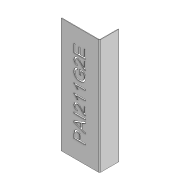
# Autodesk Inventor part: Laterales
Saved by Autodesk Inventor 2021 (Build 250183000, 183)
## iProperties
Created: 2021-04-18
Part Number: Laterales
Material: Genérico
Document SubType Name: Chapa
Designer: carlo
Density: 1 g/cm^3
Sheet Metal Rule: Por defecto_mm
Appearance: Valor por defecto
Author: carlo
Autodesk Inventor part; units mm, degrees
ref_plane "YZ Plane" through (0, 0, 0) normal (1, 0, 0) x (0, 1, 0)
ref_plane "XZ Plane" through (0, 0, 0) normal (0, 1, 0) x (-1, 0, 0)
ref_plane "XY Plane" through (0, 0, 0) normal (0, 0, 1) x (1, 0, 0)
sketch "Boceto1" plane through (0, 0, 0) normal (0, 0, 1) x (1, 0, 0)
  line L0 (0, 0) -> (200, 0)
  line L1 (200, 0) -> (200, 600)
  line L2 (200, 600) -> (0, 600)
  line L3 (0, 600) -> (0, 0)
  dimension "d0" = 200
  dimension "d1" = 600
  measures "d0" distance of L2.end L1.end
  measures "d1" distance of L1.end L0.end
extrude "Placa1" add sketch "Boceto1" along normal blind 3
sketch "Boceto2" plane through (197, 600, 3) normal (1, 0, 0) x (0, 1, 0)
  line L0 (-600, 0) -> (0, 0)
  line L1 (0, 0) -> (0, 100)
  line L2 (0, 100) -> (-600, 100)
  line L3 (-600, 100) -> (-600, 0)
  constraints: 6 end point, 1 horizontal, 1 perpendicular, 1 vertical
edge flange "Pestaña1" height 100 angle -90 thickness 3 bend radius 3 thickness toward (1, 0, 0) relief straight relief width 3 relief depth 1.5 edges at (200, 300, 3) wall of the first edge with corners at (197, 0, 3) (197, 600, 3) (197, 600, -97) (197, 0, -97)
bend "Doblez1"
corner "Esquina1"
sketch "Boceto3" plane through (0, 0, 3) normal (0, 0, 1) x (1, 0, 0)
  line L0 (65.3644, 82.3487) -> (65.3644, 522.9888) construction
  line L1 (65.3644, 522.9888) -> (130.6275, 522.9888) construction
  line L2 (130.6275, 522.9888) -> (130.6275, 82.3487) construction
  line L3 (130.6275, 82.3487) -> (65.3644, 82.3487) construction
  line L4 (0, 0) -> (0, 600) projected
  line L5 (194, 0) -> (0, 0) projected
  line L6 (0, 600) -> (194, 600) projected
  line L7 (126.4162, 88.7968) -> (66.4162, 88.7968)
  line L8 (66.4162, 88.7968) -> (66.4162, 111.434)
  spline S0 degree 2 poles (66.4162, 111.434) (66.4162, 117.4249) (67.0107, 120.5804) knots 0 0 0 1 1 1
  spline S1 degree 2 poles (67.0107, 120.5804) (67.7424, 125.0163) (71.8583, 130.9615) (79.3125, 134.62) (83.7942, 134.62) knots 0 0 0 1 2 3 3 3
  spline S2 degree 2 poles (83.7942, 134.62) (91.4314, 134.62) (102.0412, 124.8791) (102.0412, 112.1657) knots 0 0 0 1 2 2 2
  line L9 (102.0412, 112.1657) -> (102.0412, 96.7541)
  line L10 (102.0412, 96.7541) -> (126.4162, 96.7541)
  line L11 (126.4162, 96.7541) -> (126.4162, 88.7968)
  line L12 (94.9528, 96.7541) -> (94.9528, 112.2572)
  spline S3 degree 2 poles (94.9528, 112.2572) (94.9528, 119.9859) (89.2363, 126.434) (84.0229, 126.434) knots 0 0 0 1 2 2 2
  spline S4 degree 2 poles (84.0229, 126.434) (80.2729, 126.434) (74.8766, 122.6383) (74.0534, 119.5285) knots 0 0 0 1 2 2 2
  spline S5 degree 2 poles (74.0534, 119.5285) (73.5046, 117.5163) (73.5046, 112.12) knots 0 0 0 1 1 1
  line L13 (73.5046, 112.12) -> (73.5046, 96.7541)
  line L14 (73.5046, 96.7541) -> (94.9528, 96.7541)
  line L15 (126.4162, 138.1871) -> (66.4162, 161.2359)
  line L16 (66.4162, 161.2359) -> (66.4162, 169.8334)
  line L17 (66.4162, 169.8334) -> (126.4162, 194.3456)
  line L18 (126.4162, 194.3456) -> (126.4162, 185.2907)
  line L19 (126.4162, 185.2907) -> (108.2607, 178.3395)
  line L20 (108.2607, 178.3395) -> (108.2607, 153.1871)
  line L21 (108.2607, 153.1871) -> (126.4162, 146.6017)
  line L22 (126.4162, 146.6017) -> (126.4162, 138.1871)
  line L23 (101.8125, 155.4737) -> (101.8125, 175.87)
  line L24 (101.8125, 175.87) -> (85.1662, 169.559)
  spline S6 degree 2 poles (85.1662, 169.559) (77.5747, 166.7237) (72.7272, 165.3517) knots 0 0 0 1 1 1
  spline S7 degree 2 poles (72.7272, 165.3517) (78.4894, 164.1627) (84.2058, 162.1048) knots 0 0 0 1 1 1
  line L25 (84.2058, 162.1048) -> (101.8125, 155.4737)
  line L26 (126.4162, 202.0285) -> (66.4162, 202.0285)
  line L27 (66.4162, 202.0285) -> (66.4162, 209.9859)
  line L28 (66.4162, 209.9859) -> (126.4162, 209.9859)
  line L29 (126.4162, 209.9859) -> (126.4162, 202.0285)
  line L30 (119.3278, 259.6505) -> (126.4162, 259.6505)
  line L31 (126.4162, 259.6505) -> (126.4162, 220.0011)
  spline S8 degree 2 poles (126.4162, 220.0011) (123.7638, 219.9096) (121.2942, 220.87) knots 0 0 0 1 1 1
  spline S9 degree 2 poles (121.2942, 220.87) (117.2241, 222.3791) (109.404, 229.056) (104.2363, 235.367) knots 0 0 0 1 2 2 2
  spline S10 degree 2 poles (104.2363, 235.367) (96.1875, 245.1078) (86.8583, 251.9676) (82.651, 251.9676) knots 0 0 0 1 2 2 2
  spline S11 degree 2 poles (82.651, 251.9676) (78.2607, 251.9676) (72.2699, 245.7023) (72.2699, 240.6718) knots 0 0 0 1 2 2 2
  spline S12 degree 2 poles (72.2699, 240.6718) (72.2699, 235.367) (78.6723, 229.0102) (84.2973, 228.9645) knots 0 0 0 1 2 2 2
  line L32 (84.2973, 228.9645) -> (83.5199, 221.373)
  spline S13 degree 2 poles (83.5199, 221.373) (75.0595, 222.1505) (66.1875, 232.3029) (66.1875, 240.8548) knots 0 0 0 1 2 2 2
  spline S14 degree 2 poles (66.1875, 240.8548) (66.1875, 249.498) (75.7455, 259.559) (82.8339, 259.559) knots 0 0 0 1 2 2 2
  spline S15 degree 2 poles (82.8339, 259.559) (86.4467, 259.559) (93.3979, 256.6322) (101.0808, 249.7724) (107.8034, 241.8609) knots 0 0 0 1 2 3 3 3
  spline S16 degree 2 poles (107.8034, 241.8609) (113.3369, 235.2298) (117.3156, 231.4798) (119.3278, 230.245) knots 0 0 0 1 2 2 2
  line L33 (119.3278, 230.245) -> (119.3278, 259.6505)
  line L34 (126.4162, 295.2755) -> (126.4162, 287.9127)
  line L35 (126.4162, 287.9127) -> (79.4955, 287.9127)
  spline S17 degree 2 poles (79.4955, 287.9127) (82.0107, 285.2602) (87.0869, 276.617) (88.3674, 273.1871) knots 0 0 0 1 2 2 2
  line L36 (88.3674, 273.1871) -> (81.2333, 273.1871)
  spline S18 degree 2 poles (81.2333, 273.1871) (78.3522, 279.3609) (70.0747, 288.5987) (66.1875, 290.5194) knots 0 0 0 1 2 2 2
  line L37 (66.1875, 290.5194) -> (66.1875, 295.2755)
  line L38 (66.1875, 295.2755) -> (126.4162, 295.2755)
  line L39 (126.4162, 341.8761) -> (126.4162, 334.5133)
  line L40 (126.4162, 334.5133) -> (79.4955, 334.5133)
  spline S19 degree 2 poles (79.4955, 334.5133) (82.0107, 331.8609) (87.0869, 323.2176) (88.3674, 319.7877) knots 0 0 0 1 2 2 2
  line L41 (88.3674, 319.7877) -> (81.2333, 319.7877)
  spline S20 degree 2 poles (81.2333, 319.7877) (78.3522, 325.9615) (70.0747, 335.1993) (66.1875, 337.12) knots 0 0 0 1 2 2 2
  line L42 (66.1875, 337.12) -> (66.1875, 341.8761)
  line L43 (66.1875, 341.8761) -> (126.4162, 341.8761)
  line L44 (102.9101, 391.8609) -> (95.8217, 391.8609)
  line L45 (95.8217, 391.8609) -> (95.8217, 417.242)
  line L46 (95.8217, 417.242) -> (118.0473, 417.242)
  spline S21 degree 2 poles (118.0473, 417.242) (122.7119, 411.3883) (127.4223, 398.9493) (127.4223, 392.4096) knots 0 0 0 1 2 2 2
  spline S22 degree 2 poles (127.4223, 392.4096) (127.4223, 383.5834) (119.8308, 369.1322) (105.5168, 361.7694) (96.6906, 361.7694) knots 0 0 0 1 2 3 3 3
  spline S23 degree 2 poles (96.6906, 361.7694) (87.9101, 361.7694) (72.7272, 369.0865) (65.3644, 382.8517) (65.3644, 391.8151) knots 0 0 0 1 2 3 3 3
  spline S24 degree 2 poles (65.3644, 391.8151) (65.3644, 398.309) (69.5717, 408.8273) (77.1174, 414.7724) (83.1997, 416.3273) knots 0 0 0 1 2 3 3 3
  line L47 (83.1997, 416.3273) -> (85.1662, 409.1932)
  spline S25 degree 2 poles (85.1662, 409.1932) (80.593, 407.8212) (75.3339, 403.8426) (72.1784, 396.3883) (72.1784, 391.8609) knots 0 0 0 1 2 3 3 3
  spline S26 degree 2 poles (72.1784, 391.8609) (72.1784, 386.4188) (75.4711, 378.4615) (80.9131, 373.6139) (84.1144, 372.242) knots 0 0 0 1 2 3 3 3
  spline S27 degree 2 poles (84.1144, 372.242) (89.6936, 369.9554) (96.1875, 369.9554) knots 0 0 0 1 1 1
  spline S28 degree 2 poles (96.1875, 369.9554) (104.1906, 369.9554) (115.029, 375.4889) (120.2424, 386.0529) (120.2424, 391.9523) knots 0 0 0 1 2 3 3 3
  spline S29 degree 2 poles (120.2424, 391.9523) (120.2424, 397.12) (116.2638, 406.9523) (114.0229, 409.4676) knots 0 0 0 1 2 2 2
  line L48 (114.0229, 409.4676) -> (102.9101, 409.4676)
  line L49 (102.9101, 409.4676) -> (102.9101, 391.8609)
  line L50 (119.3278, 464.6657) -> (126.4162, 464.6657)
  line L51 (126.4162, 464.6657) -> (126.4162, 425.0163)
  spline S30 degree 2 poles (126.4162, 425.0163) (123.7638, 424.9249) (121.2942, 425.8852) knots 0 0 0 1 1 1
  spline S31 degree 2 poles (121.2942, 425.8852) (117.2241, 427.3944) (109.404, 434.0712) (104.2363, 440.3822) knots 0 0 0 1 2 2 2
  spline S32 degree 2 poles (104.2363, 440.3822) (96.1875, 450.123) (86.8583, 456.9828) (82.651, 456.9828) knots 0 0 0 1 2 2 2
  spline S33 degree 2 poles (82.651, 456.9828) (78.2607, 456.9828) (72.2699, 450.7176) (72.2699, 445.6871) knots 0 0 0 1 2 2 2
  spline S34 degree 2 poles (72.2699, 445.6871) (72.2699, 440.3822) (78.6723, 434.0255) (84.2973, 433.9798) knots 0 0 0 1 2 2 2
  line L52 (84.2973, 433.9798) -> (83.5199, 426.3883)
  spline S35 degree 2 poles (83.5199, 426.3883) (75.0595, 427.1657) (66.1875, 437.3182) (66.1875, 445.87) knots 0 0 0 1 2 2 2
  spline S36 degree 2 poles (66.1875, 445.87) (66.1875, 454.5133) (75.7455, 464.5743) (82.8339, 464.5743) knots 0 0 0 1 2 2 2
  spline S37 degree 2 poles (82.8339, 464.5743) (86.4467, 464.5743) (93.3979, 461.6474) (101.0808, 454.7877) (107.8034, 446.8761) knots 0 0 0 1 2 3 3 3
  spline S38 degree 2 poles (107.8034, 446.8761) (113.3369, 440.245) (117.3156, 436.495) (119.3278, 435.2602) knots 0 0 0 1 2 2 2
  line L53 (119.3278, 435.2602) -> (119.3278, 464.6657)
  line L54 (126.4162, 475.7328) -> (66.4162, 475.7328)
  line L55 (66.4162, 475.7328) -> (66.4162, 519.1779)
  line L56 (66.4162, 519.1779) -> (73.5046, 519.1779)
  line L57 (73.5046, 519.1779) -> (73.5046, 483.6901)
  line L58 (73.5046, 483.6901) -> (91.843, 483.6901)
  line L59 (91.843, 483.6901) -> (91.843, 516.9371)
  line L60 (91.843, 516.9371) -> (98.9314, 516.9371)
  line L61 (98.9314, 516.9371) -> (98.9314, 483.6901)
  line L62 (98.9314, 483.6901) -> (119.3278, 483.6901)
  line L63 (119.3278, 483.6901) -> (119.3278, 520.5499)
  line L64 (119.3278, 520.5499) -> (126.4162, 520.5499)
  line L65 (126.4162, 520.5499) -> (126.4162, 475.7328)
  constraints: 1 parallel, 2 other
emboss "Repujado1" sketch "Boceto3" operation cut depth 3 direction (0, 0, -1)
equation "\"d2\" = Grosor"
equation "\"d3\" = Anchura_desahogo_plegado"
equation "\"d4\" = Profundidad_desahogo_plegado"
equation "\"d5\" = Remanente_mínimo"
equation "\"d6\" = Radiodetransición"
equation "\"d9\" = Radio_pliegue"
equation "\"d10\" = Tamaño_destalonado"
equation "\"d11\" = TamañoSeparación"
equation "\"d12\" = Tamaño_de_radio_de_Jacobi"
equation "\"Radio_pliegue\" = Grosor"
equation "\"Anchura_desahogo_plegado\" = Grosor"
equation "\"Profundidad_desahogo_plegado\" = 0.5 * Grosor"
equation "\"Tamaño_destalonado\" = 4 * Grosor"
equation "\"Remanente_mínimo\" = 2 * Grosor"
equation "\"Radiodetransición\" = Radio_pliegue"
equation "\"Tamaño_de_radio_de_Jacobi\" = Radio_pliegue"
equation "\"TamañoSeparación\" = Grosor"
equation "\"Grosor\" = 3"
